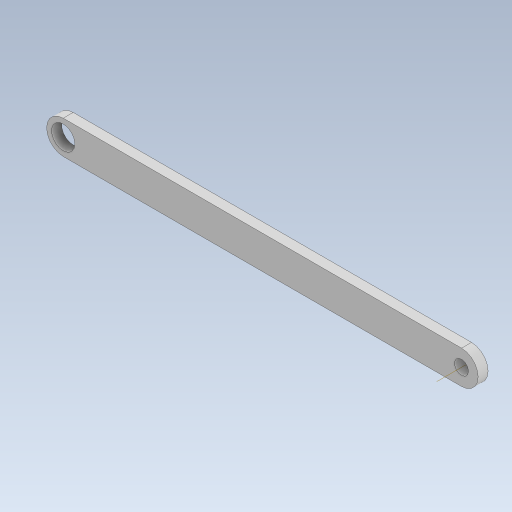
# Autodesk Inventor part: adjustable_120
Saved by Autodesk Inventor 2023 (Build 270158000, 158)
## iProperties
Created: 2023-04-16
Part Number: adjustable_120
Material: 一般
Document SubType Name: Modeling
Designer: JOU
Density: 1 g/cm^3
Appearance: 預設
Author: JOU
Autodesk Inventor part; units mm, degrees
ref_plane "YZ Plane" through (0, 0, 0) normal (1, 0, 0) x (0, 1, 0)
ref_plane "XZ Plane" through (0, 0, 0) normal (0, 1, 0) x (-1, 0, 0)
ref_plane "XY Plane" through (0, 0, 0) normal (0, 0, 1) x (1, 0, 0)
sketch "草圖1" plane through (0, 0, 0) normal (0, 0, 1) x (1, 0, 0)
  line L0 (-120, 0) -> (0, 0) construction
  line L1 (-120, -5) -> (0, -5)
  line L2 (0, 5) -> (-120, 5)
  arc A0 (-120, 5) -> (-120, -5) centre (-120, 0) ccw
  arc A1 (0, -5) -> (0, 5) centre (0, 0) ccw
  circle A2 centre (-120, 0) radius 3.5
  circle A3 centre (0, 0) radius 2.1
  point P0 (-60, 0)
  dimension "d0" = 120
  dimension "d1" = 10
  dimension "d2" = 7
  dimension "d3" = 4.2
  constraints: 8 end point, 4 centre point, 4 point on circle, 4 tangent, 3 coincident, 1 horizontal, 1 midpoint, 1 parallel
  measures "d0" distance of L2.start L2.end
  measures "d1" distance between parallel lines of L1 L2
  measures "d2" diameter of A2
  measures "d3" diameter of A3
extrude "擠出1" add sketch "草圖1" along normal blind 3
sketch "草圖4" plane through (0, 0, 3) normal (0, 0, 1) x (1, 0, 0)
  line L0 (2.932, 0.7895) -> (0.36, 2.1968)
  arc A0 (0.36, 2.1968) -> (-0.36, 2.1968) centre (0, 1.5389) ccw
  line L1 (-0.36, 2.1968) -> (-2.932, 0.7895)
  arc A1 (-2.932, 0.7895) -> (-2.932, -0.7895) centre (-2.5, 0) ccw
  line L2 (-2.932, -0.7895) -> (-0.36, -2.1968)
  arc A2 (-0.36, -2.1968) -> (0.36, -2.1968) centre (0, -1.5389) ccw
  line L3 (0.36, -2.1968) -> (2.932, -0.7895)
  arc A3 (2.932, -0.7895) -> (2.932, 0.7895) centre (2.5, 0) ccw
  circle A4 centre (0, 0) radius 1.55
  constraints: 8 end point, 8 point on circle, 5 centre point
extrude "擠出3" [suppressed]
